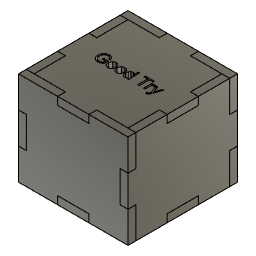
Box V2 v3 (Autodesk Fusion 360 design; units mm, degrees)
Autodesk Fusion 360 part; units mm, degrees
note: some values were not read from the file. Chosen so that the rebuilt part matches the saved one: which bodies a step acts on; the layout of a text.
sketch "Top-Bottom" plane through (0, 0, 0) normal (0, 0, 1) x (1, 0, 0)
  line L0 (0, 0) -> (30, 0)
  line L1 (30, 0) -> (30, 30)
  line L2 (30, 30) -> (0, 30)
  line L3 (0, 30) -> (0, 0)
  line L4 (-2.5, 20) -> (0, 20)
  line L5 (0, 20) -> (0, 10)
  line L6 (0, 10) -> (-2.5, 10)
  line L7 (-2.5, 10) -> (-2.5, 20)
  line L8 (15, 30) -> (15, 0) construction
  line L9 (0, 15) -> (30, 15) construction
  line L10 (10, 32.5) -> (20, 32.5)
  line L11 (20, 32.5) -> (20, 30)
  line L12 (20, 30) -> (10, 30)
  line L13 (10, 30) -> (10, 32.5)
  line L14 (20, 0) -> (10, 0)
  line L15 (10, 0) -> (10, -2.5)
  line L16 (20, -2.5) -> (20, 0)
  line L17 (10, -2.5) -> (20, -2.5)
  line L18 (30, 20) -> (30, 10)
  line L19 (30, 10) -> (32.5, 10)
  line L20 (32.5, 20) -> (30, 20)
  line L21 (32.5, 10) -> (32.5, 20)
  point P0 (15, 0)
  point P1 (30, 15)
  dimension "d4" = 30
  dimension "d5" = 30
  dimension "d9" = 2.5
  dimension "d10" = 10
  dimension "d11" = 10
  dimension "d12" = 2.5
  constraint horizontal L0
  constraint vertical L1
  constraint horizontal L2
  constraint vertical L3
  constraint coincident L0.start L3.end
  constraint horizontal L4
  constraint vertical L5
  constraint horizontal L6
  constraint vertical L7
  constraint midpoint L3 L5
  constraint midpoint L2 L8.start
  constraint midpoint L0 P0
  constraint midpoint L3 L9.start
  constraint midpoint L1 P1
  constraint horizontal L10
  constraint vertical L11
  constraint horizontal L12
  constraint vertical L13
  constraint midpoint L2 L12
  constraint symmetric L8.start L9 P0
  constraint symmetric L9 L10.start L15.end
  constraint symmetric L9 L10.end L16.start
  constraint symmetric L9 L11.end L14.start
  constraint symmetric L9 L12.end L14.end
  constraint symmetric L4.start L8 L20.start
  constraint symmetric L4.end L8 L18.start
  constraint symmetric L5.end L8 L18.end
  constraint symmetric L6.end L8 L19.end
  constraint symmetric L8 L9.start P1
  measures "d4" distance of L0.start L0.end
  measures "d5" distance of L0.start L2.end
  measures "d9" distance of L4.start L4.end
  measures "d10" distance of L4.start L6.end
  measures "d11" distance of L10.start L10.end
  measures "d12" distance of L10.start L12.end
extrude "Extrude1" add sketch "Top-Bottom" along normal blind 2.5 makes body 1
sketch "Front-Back" plane through (0, -2.5, 0) normal (0, -1, 0) x (1, 0, 0)
  line L0 (10, 0) -> (20, 0)
  line L1 (20, 0) -> (20, 2.5)
  line L2 (20, 2.5) -> (10, 2.5)
  line L3 (10, 2.5) -> (10, 0)
  line L4 (0, 0) -> (30, 0)
  line L5 (30, 0) -> (30, 30)
  line L6 (30, 30) -> (0, 30)
  line L7 (0, 30) -> (0, 0)
  line L8 (-2.5, 10) -> (0, 10)
  line L9 (0, 10) -> (0, 0)
  line L10 (0, 0) -> (-2.5, 0)
  line L11 (-2.5, 0) -> (-2.5, 10)
  line L12 (0, 20) -> (-2.5, 20)
  line L13 (-2.5, 30) -> (0, 30)
  line L14 (0, 30) -> (0, 20)
  line L15 (-2.5, 20) -> (-2.5, 30)
  line L16 (15, 30) -> (15, 0) construction
  line L17 (32.5, 30) -> (30, 30)
  line L18 (30, 20) -> (32.5, 20)
  line L19 (32.5, 20) -> (32.5, 30)
  line L20 (30, 30) -> (30, 20)
  line L21 (32.5, 0) -> (32.5, 10)
  line L22 (30, 0) -> (32.5, 0)
  line L23 (32.5, 10) -> (30, 10)
  line L24 (30, 10) -> (30, 0)
  point P0 (30, 30)
  point P1 (30, 0)
  point P2 (30, 0)
  dimension "d18" = 30
  dimension "d19" = 30
  dimension "d20" = 2.5
  dimension "d21" = 10
  dimension "d22" = 2.5
  dimension "d23" = 10
  constraint horizontal L4
  constraint vertical L5
  constraint horizontal L6
  constraint vertical L7
  constraint coincident L4.start L7.end
  constraint horizontal L8
  constraint vertical L9
  constraint horizontal L10
  constraint vertical L11
  constraint horizontal L13
  constraint vertical L14
  constraint horizontal L12
  constraint vertical L15
  constraint coincident L6.end L7.start
  constraint midpoint L6 L16.start
  constraint midpoint L4 L16.end
  constraint symmetric L4.start L16 P2
  constraint symmetric L6.end L16 P0
  constraint symmetric L8.start L16 L21.end
  constraint symmetric L8.end L16 L23.end
  constraint symmetric L10.end L16 L21.start
  constraint symmetric L13.start L16 L17.start
  constraint symmetric L12.start L16 L18.start
  constraint symmetric L12.end L16 L18.end
  measures "d18" distance of L4.start P2
  measures "d19" distance of L4.start L6.end
  measures "d20" distance of L8.start L8.end
  measures "d21" distance of L8.start L10.end
  measures "d22" distance of L13.start L6.end
  measures "d23" distance of L13.start L12.end
extrude "Extrude2" add sketch "Front-Back" against normal blind 2.5 separate body contours L1 L2 L3 L4 L5 L6 L7 L9 L14 L20 L24 | L7 L8 L9 L10 L11 | L5 L21 L22 L23 L24 | L7 L12 L13 L14 L15 | L5 L17 L18 L19 L20 makes body 2
ref_plane "WorkPlane1" through (15, 15, 15) normal (0, 0, -1) x (-1, 0, 0)
mirror "Mirror1" about plane through (15, 15, 15) normal (0, 0, -1) of bodies 1 makes body 3
ref_plane "WorkPlane2" through (15, 15, 15) normal (0, 1, 0) x (0, 0, 1)
mirror "Mirror2" about plane through (15, 15, 15) normal (0, 1, 0) of bodies 2 makes body 4
combine "Combine1" operation cut target body 2 tool bodies 3 keep tools
combine "Combine2" operation cut target body 4 tool bodies 3 keep tools
sketch "Left-Right" plane through (32.5, 0, 0) normal (1, 0, 0) x (0, 1, 0)
  line L0 (10, 0) -> (20, 0)
  line L1 (20, 0) -> (20, 2.5)
  line L2 (20, 2.5) -> (10, 2.5)
  line L3 (10, 2.5) -> (10, 0)
  line L4 (0, 0) -> (30, 0)
  line L5 (30, 0) -> (30, 30)
  line L6 (30, 30) -> (0, 30)
  line L7 (0, 30) -> (0, 0)
  line L8 (-2.5, 20) -> (0, 20)
  line L9 (0, 20) -> (0, 10)
  line L10 (0, 10) -> (-2.5, 10)
  line L11 (-2.5, 10) -> (-2.5, 20)
  line L12 (15, 30) -> (15, 0) construction
  line L13 (30, 10) -> (32.5, 10)
  line L14 (30, 20) -> (30, 10)
  line L15 (32.5, 10) -> (32.5, 20)
  line L16 (32.5, 20) -> (30, 20)
  dimension "d30" = 30
  dimension "d31" = 30
  dimension "d32" = 2.5
  dimension "d33" = 10
  constraint horizontal L4
  constraint vertical L5
  constraint horizontal L6
  constraint vertical L7
  constraint coincident L4.start L7.end
  constraint horizontal L8
  constraint vertical L9
  constraint horizontal L10
  constraint vertical L11
  constraint midpoint L7 L9
  constraint midpoint L6 L12.start
  constraint midpoint L4 L12.end
  constraint symmetric L8.start L12 L15.end
  constraint symmetric L8.end L12 L14.start
  constraint symmetric L9.end L12 L13.start
  constraint symmetric L10.end L12 L13.end
  measures "d30" distance of L4.start L4.end
  measures "d31" distance of L4.start L6.end
  measures "d32" distance of L8.start L8.end
  measures "d33" distance of L8.start L10.end
extrude "Extrude3" add sketch "Left-Right" against normal blind 2.5 separate body contours L1 L2 L3 L4 L5 L6 L7 L9 L14 | L7 L8 L9 L10 L11 | L5 L13 L14 L15 L16 makes body 5
combine "Combine3" operation cut target body 5 tool bodies 3 keep tools
ref_plane "WorkPlane3" through (15, 15, 15) normal (-1, 0, 0) x (0, 0, 1)
mirror "Mirror3" about plane through (15, 15, 15) normal (-1, 0, 0) of bodies 5 makes body 6
sketch "Text-Top" plane through (0, 0, 30) normal (0, 0, 1) x (-1, 0, 0)
  line L0 (0, -10) -> (0, 0)
  line L1 (0, 0) -> (-10, 0)
  line L2 (-10, 0) -> (-10, 2.5)
  line L3 (-10, 2.5) -> (-20, 2.5)
  line L4 (-20, 2.5) -> (-20, 0)
  line L5 (-20, 0) -> (-30, 0)
  line L6 (-30, 0) -> (-30, -10)
  line L7 (-30, -10) -> (-32.5, -10)
  line L8 (-32.5, -10) -> (-32.5, -20)
  line L9 (-32.5, -20) -> (-30, -20)
  line L10 (-30, -20) -> (-30, -30)
  line L11 (-30, -30) -> (-20, -30)
  line L12 (-20, -30) -> (-20, -32.5)
  line L13 (-20, -32.5) -> (-10, -32.5)
  line L14 (-10, -32.5) -> (-10, -30)
  line L15 (-10, -30) -> (0, -30)
  line L16 (0, -30) -> (0, -20)
  line L17 (0, -20) -> (2.5, -20)
  line L18 (2.5, -20) -> (2.5, -10)
  line L19 (2.5, -10) -> (0, -10)
  line L20 (-5, -12.5) -> (-25, -12.5) construction
  line L21 (-25, -12.5) -> (-25, -17.5) construction
  line L22 (-25, -17.5) -> (-5, -17.5) construction
  line L23 (-5, -17.5) -> (-5, -12.5) construction
  line L24 (2.5, -15) -> (-5, -15) construction
  line L25 (-25, -15) -> (-32.5, -15) construction
  dimension "d39" = 5
  dimension "d42" = 7.5
  dimension "d43" = 7.5
  text T0 "Good Try" font "Arial" height 5 align ink ink in box 0 x 0 at (-5.01, -12.52) x (-1, 0) y (0, -1) spacing 1 kerned height is em
  constraint perpendicular L20 L21
  constraint parallel L20 L22
  constraint parallel L21 L23
  constraint midpoint L18 L24.start
  constraint perpendicular L18 L24
  constraint midpoint L23 L24.end
  constraint midpoint L21 L25.start
  constraint midpoint L8 L25.end
  constraint perpendicular L8 L25
  measures "d39" distance of L20.end L21.end
  measures "d42" distance of L24.start L24.end
  measures "d43" distance of L25.start L25.end
extrude "Extrude4" cut sketch "Text-Top" against normal blind 2.5 text T0 bodies 3 makes body 7 at (12.6268, 15.5251, 30) makes body 8 at (15.3464, 15.5191, 30) makes body 9 at (15.1604, 4.5046, 30)
delete_body "RemoveBody1" bodies 3
delete_body "RemoveBody2" bodies 7
delete_body "RemoveBody3" bodies 8
sketch "Final-Top" plane through (0, 0, 30) normal (0, 0, 1) x (-1, 0, 0)
  line L0 (0, -10) -> (0, 0)
  line L1 (0, 0) -> (-10, 0)
  line L2 (-10, 0) -> (-10, 2.5)
  line L3 (-10, 2.5) -> (-20, 2.5)
  line L4 (-20, 2.5) -> (-20, 0)
  line L5 (-20, 0) -> (-30, 0)
  line L6 (-30, 0) -> (-30, -10)
  line L7 (-30, -10) -> (-32.5, -10)
  line L8 (-32.5, -10) -> (-32.5, -20)
  line L9 (-32.5, -20) -> (-30, -20)
  line L10 (-30, -20) -> (-30, -30)
  line L11 (-30, -30) -> (-20, -30)
  line L12 (-20, -30) -> (-20, -32.5)
  line L13 (-20, -32.5) -> (-10, -32.5)
  line L14 (-10, -32.5) -> (-10, -30)
  line L15 (-10, -30) -> (0, -30)
  line L16 (0, -30) -> (0, -20)
  line L17 (0, -20) -> (2.5, -20)
  line L18 (2.5, -20) -> (2.5, -10)
  line L19 (2.5, -10) -> (0, -10)
  line L20 (-7.8567, -14.3096) -> (-7.8567, -14.9761)
  line L21 (-7.8567, -14.9761) -> (-6.8044, -14.9761)
  line L22 (-6.8044, -14.9761) -> (-6.8044, -15.396)
  line L23 (-6.8044, -15.396) -> (-8.3205, -15.3984)
  line L24 (-8.3205, -15.3984) -> (-8.3205, -14.0703)
  spline S0 degree 3 poles (-8.3205, -14.0703) (-8.2052, -13.984) (-7.9813, -13.8165) (-7.7248, -13.7055) (-7.6003, -13.6516) knots 0 0 0 0 0.043036 0.083562 0.083562 0.083562 0.083562
  spline S1 degree 3 poles (-7.6003, -13.6516) (-7.4761, -13.6106) (-7.2286, -13.5291) (-6.9683, -13.5172) (-6.8386, -13.5112) knots 0 0 0 0 0.039044 0.077778 0.077778 0.077778 0.077778
  spline S2 degree 3 poles (-6.8386, -13.5112) (-6.6684, -13.5198) (-6.3351, -13.5366) (-6.0298, -13.6712) (-5.8804, -13.737) knots 0 0 0 0 0.050639 0.099191 0.099191 0.099191 0.099191
  spline S3 degree 3 poles (-5.8804, -13.737) (-5.7456, -13.8205) (-5.4771, -13.9868) (-5.312, -14.256) (-5.2297, -14.3901) knots 0 0 0 0 0.046824 0.093334 0.093334 0.093334 0.093334
  spline S4 degree 3 poles (-5.2297, -14.3901) (-5.1657, -14.5387) (-5.0343, -14.8434) (-5.0182, -15.1749) (-5.01, -15.3447) knots 0 0 0 0 0.048136 0.098667 0.098667 0.098667 0.098667
  spline S5 degree 3 poles (-5.01, -15.3447) (-5.0187, -15.5152) (-5.036, -15.8528) (-5.1648, -16.1653) (-5.2285, -16.32) knots 0 0 0 0 0.050801 0.100602 0.100602 0.100602 0.100602
  spline S6 degree 3 poles (-5.2285, -16.32) (-5.3078, -16.4605) (-5.4633, -16.7356) (-5.7277, -16.9082) (-5.8572, -16.9927) knots 0 0 0 0 0.047611 0.093274 0.093274 0.093274 0.093274
  spline S7 degree 3 poles (-5.8572, -16.9927) (-6.0021, -17.0567) (-6.3029, -17.1897) (-6.6316, -17.2046) (-6.802, -17.2124) knots 0 0 0 0 0.047105 0.097758 0.097758 0.097758 0.097758
  spline S8 degree 3 poles (-6.802, -17.2124) (-6.9263, -17.2079) (-7.1663, -17.1993) (-7.3941, -17.1233) (-7.5039, -17.0867) knots 0 0 0 0 0.03709 0.071636 0.071636 0.071636 0.071636
  spline S9 degree 3 poles (-7.5039, -17.0867) (-7.6014, -17.0424) (-7.7884, -16.9575) (-7.9287, -16.8079) (-7.9958, -16.7363) knots 0 0 0 0 0.031773 0.060917 0.060917 0.060917 0.060917
  spline S10 degree 3 poles (-7.9958, -16.7363) (-8.0526, -16.6521) (-8.1743, -16.4716) (-8.2346, -16.2622) (-8.2668, -16.1504) knots 0 0 0 0 0.030262 0.06491 0.06491 0.06491 0.06491
  line L25 (-8.2668, -16.1504) -> (-7.8396, -16.0332)
  spline S11 degree 3 poles (-7.8396, -16.0332) (-7.8133, -16.1164) (-7.7653, -16.2685) (-7.6787, -16.4023) (-7.6394, -16.4629) knots 0 0 0 0 0.026032 0.047595 0.047595 0.047595 0.047595
  spline S12 degree 3 poles (-7.6394, -16.4629) (-7.5934, -16.5131) (-7.4964, -16.6192) (-7.3662, -16.6807) (-7.2976, -16.7131) knots 0 0 0 0 0.020222 0.042723 0.042723 0.042723 0.042723
  spline S13 degree 3 poles (-7.2976, -16.7131) (-7.2202, -16.7405) (-7.0607, -16.797) (-6.8916, -16.8037) (-6.8044, -16.8071) knots 0 0 0 0 0.024475 0.05046 0.05046 0.05046 0.05046
  spline S14 degree 3 poles (-6.8044, -16.8071) (-6.7026, -16.8041) (-6.5104, -16.7984) (-6.3284, -16.737) (-6.2429, -16.7082) knots 0 0 0 0 0.030374 0.057295 0.057295 0.057295 0.057295
  spline S15 degree 3 poles (-6.2429, -16.7082) (-6.1689, -16.6739) (-6.0272, -16.6082) (-5.9147, -16.5) (-5.8608, -16.4482) knots 0 0 0 0 0.024261 0.046502 0.046502 0.046502 0.046502
  spline S16 degree 3 poles (-5.8608, -16.4482) (-5.8152, -16.3935) (-5.7249, -16.2851) (-5.6648, -16.1574) (-5.635, -16.0942) knots 0 0 0 0 0.021272 0.042143 0.042143 0.042143 0.042143
  spline S17 degree 3 poles (-5.635, -16.0942) (-5.5951, -15.98) (-5.5138, -15.7468) (-5.5035, -15.4999) (-5.4983, -15.374) knots 0 0 0 0 0.036094 0.073664 0.073664 0.073664 0.073664
  spline S18 degree 3 poles (-5.4983, -15.374) (-5.5029, -15.2256) (-5.5116, -14.9487) (-5.6151, -14.6922) (-5.6631, -14.5732) knots 0 0 0 0 0.044138 0.082326 0.082326 0.082326 0.082326
  spline S19 degree 3 poles (-5.6631, -14.5732) (-5.7238, -14.4729) (-5.8444, -14.2739) (-6.0439, -14.1541) (-6.1428, -14.0947) knots 0 0 0 0 0.034607 0.068675 0.068675 0.068675 0.068675
  spline S20 degree 3 poles (-6.1428, -14.0947) (-6.2495, -14.0491) (-6.4633, -13.9578) (-6.6955, -13.9449) (-6.8118, -13.9385) knots 0 0 0 0 0.034521 0.069165 0.069165 0.069165 0.069165
  spline S21 degree 3 poles (-6.8118, -13.9385) (-6.914, -13.9435) (-7.12, -13.9537) (-7.3144, -14.0223) (-7.4123, -14.0569) knots 0 0 0 0 0.030539 0.061503 0.061503 0.061503 0.061503
  spline S22 degree 3 poles (-7.4123, -14.0569) (-7.5004, -14.0939) (-7.6588, -14.1604) (-7.7958, -14.2637) (-7.8567, -14.3096) knots 0 0 0 0 0.028516 0.05129 0.05129 0.05129 0.05129
  spline S23 degree 3 poles (-12.7956, -13.5137) (-12.6249, -13.5262) (-12.2942, -13.5504) (-12.0389, -13.761) (-11.9155, -13.8628) knots 0 0 0 0 0.049993 0.096791 0.096791 0.096791 0.096791
  spline S24 degree 3 poles (-11.9155, -13.8628) (-11.8178, -13.9999) (-11.6044, -14.2994) (-11.5884, -14.6685) (-11.5798, -14.8686) knots 0 0 0 0 0.049486 0.108074 0.108074 0.108074 0.108074
  spline S25 degree 3 poles (-11.5798, -14.8686) (-11.5898, -15.0869) (-11.6083, -15.4883) (-11.8637, -15.7954) (-11.9802, -15.9355) knots 0 0 0 0 0.063477 0.116753 0.116753 0.116753 0.116753
  spline S26 degree 3 poles (-11.9802, -15.9355) (-12.0996, -16.0195) (-12.3442, -16.1916) (-12.6428, -16.2128) (-12.7956, -16.2236) knots 0 0 0 0 0.042941 0.087955 0.087955 0.087955 0.087955
  spline S27 degree 3 poles (-12.7956, -16.2236) (-12.9642, -16.2106) (-13.2927, -16.1852) (-13.5462, -15.9754) (-13.6697, -15.8733) knots 0 0 0 0 0.049367 0.096242 0.096242 0.096242 0.096242
  spline S28 degree 3 poles (-13.6697, -15.8733) (-13.7685, -15.7393) (-13.9801, -15.4527) (-13.999, -15.0955) (-14.009, -14.9053) knots 0 0 0 0 0.048869 0.104602 0.104602 0.104602 0.104602
  spline S29 degree 3 poles (-14.009, -14.9053) (-14.0061, -14.7543) (-14.0008, -14.4827) (-13.9025, -14.2301) (-13.8589, -14.1179) knots 0 0 0 0 0.044866 0.080708 0.080708 0.080708 0.080708
  spline S30 degree 3 poles (-13.8589, -14.1179) (-13.803, -14.0275) (-13.6908, -13.8462) (-13.5117, -13.7304) (-13.4219, -13.6723) knots 0 0 0 0 0.03145 0.063109 0.063109 0.063109 0.063109
  spline S31 degree 3 poles (-13.4219, -13.6723) (-13.3236, -13.6261) (-13.1251, -13.5326) (-12.9061, -13.52) (-12.7956, -13.5137) knots 0 0 0 0 0.032274 0.065137 0.065137 0.065137 0.065137
  line L26 (-16.614, -17.1513) -> (-16.614, -13.5722)
  line L27 (-16.614, -13.5722) -> (-16.2063, -13.5722)
  line L28 (-16.2063, -13.5722) -> (-16.2063, -13.8994)
  spline S32 degree 3 poles (-16.2063, -13.8994) (-16.1134, -13.7869) (-15.9251, -13.5588) (-15.6305, -13.5288) (-15.4812, -13.5137) knots 0 0 0 0 0.042007 0.085152 0.085152 0.085152 0.085152
  spline S33 degree 3 poles (-15.4812, -13.5137) (-15.3799, -13.5208) (-15.1771, -13.5351) (-14.9998, -13.6347) (-14.9111, -13.6846) knots 0 0 0 0 0.03006 0.060176 0.060176 0.060176 0.060176
  spline S34 degree 3 poles (-14.9111, -13.6846) (-14.8288, -13.7482) (-14.6606, -13.8785) (-14.5598, -14.066) (-14.5083, -14.1618) knots 0 0 0 0 0.030848 0.063081 0.063081 0.063081 0.063081
  spline S35 degree 3 poles (-14.5083, -14.1618) (-14.4667, -14.2704) (-14.3797, -14.497) (-14.3703, -14.7397) (-14.3655, -14.8662) knots 0 0 0 0 0.034627 0.072303 0.072303 0.072303 0.072303
  spline S36 degree 3 poles (-14.3655, -14.8662) (-14.3701, -14.9907) (-14.3791, -15.2319) (-14.4571, -15.4602) (-14.4949, -15.5705) knots 0 0 0 0 0.037159 0.071956 0.071956 0.071956 0.071956
  spline S37 degree 3 poles (-14.4949, -15.5705) (-14.5422, -15.669) (-14.6343, -15.8606) (-14.8016, -15.9915) (-14.883, -16.0552) knots 0 0 0 0 0.03227 0.062841 0.062841 0.062841 0.062841
  spline S38 degree 3 poles (-14.883, -16.0552) (-14.9723, -16.1043) (-15.1526, -16.2035) (-15.358, -16.2169) (-15.4617, -16.2236) knots 0 0 0 0 0.030177 0.060923 0.060923 0.060923 0.060923
  spline S39 degree 3 poles (-15.4617, -16.2236) (-15.5366, -16.22) (-15.6821, -16.2131) (-15.8148, -16.1536) (-15.8791, -16.1247) knots 0 0 0 0 0.022293 0.043242 0.043242 0.043242 0.043242
  spline S40 degree 3 poles (-15.8791, -16.1247) (-15.937, -16.0897) (-16.051, -16.0208) (-16.1354, -15.9178) (-16.177, -15.8672) knots 0 0 0 0 0.020129 0.039633 0.039633 0.039633 0.039633
  line L29 (-16.177, -15.8672) -> (-16.177, -17.1513)
  line L30 (-16.177, -17.1513) -> (-16.614, -17.1513)
  line L31 (-21.907, -14.9297) -> (-21.907, -13.5722)
  line L32 (-21.907, -13.5722) -> (-21.4675, -13.5722)
  line L33 (-21.4675, -13.5722) -> (-21.4675, -16.165)
  line L34 (-21.4675, -16.165) -> (-21.863, -16.165)
  line L35 (-21.863, -16.165) -> (-21.863, -15.772)
  spline S41 degree 3 poles (-21.863, -15.772) (-21.9071, -15.8518) (-21.982, -15.9877) (-22.0957, -16.0925) (-22.1426, -16.1357) knots 0 0 0 0 0.027125 0.046136 0.046136 0.046136 0.046136
  spline S42 degree 3 poles (-22.1426, -16.1357) (-22.1863, -16.1614) (-22.2735, -16.2125) (-22.3743, -16.2199) (-22.4246, -16.2236) knots 0 0 0 0 0.014986 0.029889 0.029889 0.029889 0.029889
  spline S43 degree 3 poles (-22.4246, -16.2236) (-22.5007, -16.2166) (-22.6611, -16.2018) (-22.8021, -16.1233) (-22.8762, -16.082) knots 0 0 0 0 0.022678 0.047799 0.047799 0.047799 0.047799
  line L36 (-22.8762, -16.082) -> (-22.7248, -15.6743)
  spline S44 degree 3 poles (-22.7248, -15.6743) (-22.6723, -15.7021) (-22.5711, -15.7555) (-22.4573, -15.765) (-22.4026, -15.7695) knots 0 0 0 0 0.017625 0.033913 0.033913 0.033913 0.033913
  spline S45 degree 3 poles (-22.4026, -15.7695) (-22.3558, -15.7659) (-22.2623, -15.7587) (-22.1833, -15.7081) (-22.1438, -15.6828) knots 0 0 0 0 0.013843 0.027672 0.027672 0.027672 0.027672
  spline S46 degree 3 poles (-22.1438, -15.6828) (-22.1081, -15.6504) (-22.0343, -15.5835) (-21.9986, -15.4904) (-21.9802, -15.4424) knots 0 0 0 0 0.014269 0.029448 0.029448 0.029448 0.029448
  spline S47 degree 3 poles (-21.9802, -15.4424) (-21.9589, -15.361) (-21.9147, -15.193) (-21.9096, -15.0193) (-21.907, -14.9297) knots 0 0 0 0 0.025144 0.05194 0.05194 0.05194 0.05194
  line L37 (-20.0442, -16.729) -> (-20.0442, -13.5722)
  line L38 (-20.0442, -13.5722) -> (-19.5705, -13.5722)
  line L39 (-19.5705, -13.5722) -> (-19.5705, -16.729)
  line L40 (-19.5705, -16.729) -> (-18.3913, -16.729)
  line L41 (-18.3913, -16.729) -> (-18.3913, -17.1513)
  line L42 (-18.3913, -17.1513) -> (-21.2283, -17.1513)
  line L43 (-21.2283, -17.1513) -> (-21.2283, -16.729)
  line L44 (-21.2283, -16.729) -> (-20.0442, -16.729)
  spline S48 degree 3 poles (-23.7624, -12.6213) (-23.7083, -12.5918) (-23.5958, -12.5304) (-23.4676, -12.5235) (-23.4011, -12.52) knots 0 0 0 0 0.018258 0.037953 0.037953 0.037953 0.037953
  spline S49 degree 3 poles (-23.4011, -12.52) (-23.356, -12.5228) (-23.2594, -12.5287) (-23.1671, -12.5581) (-23.1179, -12.5737) knots 0 0 0 0 0.013495 0.028922 0.028922 0.028922 0.028922
  line L45 (-23.1179, -12.5737) -> (-23.0691, -12.9863)
  spline S50 degree 3 poles (-23.0691, -12.9863) (-23.1138, -12.9749) (-23.1964, -12.9539) (-23.2815, -12.9493) (-23.3205, -12.9472) knots 0 0 0 0 0.013803 0.025502 0.025502 0.025502 0.025502
  spline S51 degree 3 poles (-23.3205, -12.9472) (-23.3651, -12.9484) (-23.4464, -12.9504) (-23.5212, -12.9819) (-23.5549, -12.9961) knots 0 0 0 0 0.01324 0.024128 0.024128 0.024128 0.024128
  spline S52 degree 3 poles (-23.5549, -12.9961) (-23.583, -13.0141) (-23.6397, -13.0505) (-23.6791, -13.1052) (-23.699, -13.1328) knots 0 0 0 0 0.009913 0.020017 0.020017 0.020017 0.020017
  spline S53 degree 3 poles (-23.699, -13.1328) (-23.7176, -13.1708) (-23.7697, -13.2767) (-23.8084, -13.3884) (-23.8332, -13.4599) knots 0 0 0 0 0.012695 0.035391 0.035391 0.035391 0.035391
  spline S54 degree 3 poles (-23.8332, -13.4599) (-23.8385, -13.475) (-23.851, -13.511) (-23.8645, -13.5467) (-23.8723, -13.5674) knots 0 0 0 0 0.004787 0.011431 0.011431 0.011431 0.011431
  line L46 (-23.8723, -13.5674) -> (-22.8884, -16.165)
  line L47 (-22.8884, -16.165) -> (-23.3621, -16.165)
  line L48 (-23.3621, -16.165) -> (-23.9016, -14.6636)
  spline S55 degree 3 poles (-23.9016, -14.6636) (-23.9359, -14.5663) (-24.0057, -14.3683) (-24.0613, -14.1659) (-24.0896, -14.063) knots 0 0 0 0 0.03094 0.06295 0.06295 0.06295 0.06295
  spline S56 degree 3 poles (-24.0896, -14.063) (-24.116, -14.1631) (-24.1685, -14.3624) (-24.2364, -14.5569) (-24.2703, -14.6538) knots 0 0 0 0 0.031038 0.061804 0.061804 0.061804 0.061804
  line L49 (-24.2703, -14.6538) -> (-24.8245, -16.165)
  line L50 (-24.8245, -16.165) -> (-25.2639, -16.165)
  line L51 (-25.2639, -16.165) -> (-24.2776, -13.5283)
  spline S57 degree 3 poles (-24.2776, -13.5283) (-24.2328, -13.4071) (-24.159, -13.2074) (-24.0671, -13.0154) (-24.031, -12.9399) knots 0 0 0 0 0.038729 0.063825 0.063825 0.063825 0.063825
  spline S58 degree 3 poles (-24.031, -12.9399) (-23.9928, -12.8739) (-23.922, -12.7516) (-23.8128, -12.6624) (-23.7624, -12.6213) knots 0 0 0 0 0.022641 0.041975 0.041975 0.041975 0.041975
  spline S59 degree 3 poles (-10.0149, -13.5137) (-9.8441, -13.5262) (-9.5134, -13.5504) (-9.2582, -13.761) (-9.1348, -13.8628) knots 0 0 0 0 0.049993 0.096791 0.096791 0.096791 0.096791
  spline S60 degree 3 poles (-9.1348, -13.8628) (-9.037, -13.9999) (-8.8236, -14.2994) (-8.8077, -14.6685) (-8.7991, -14.8686) knots 0 0 0 0 0.049486 0.108074 0.108074 0.108074 0.108074
  spline S61 degree 3 poles (-8.7991, -14.8686) (-8.8091, -15.0869) (-8.8275, -15.4883) (-9.0829, -15.7954) (-9.1995, -15.9355) knots 0 0 0 0 0.063477 0.116753 0.116753 0.116753 0.116753
  spline S62 degree 3 poles (-9.1995, -15.9355) (-9.3189, -16.0195) (-9.5634, -16.1916) (-9.8621, -16.2128) (-10.0149, -16.2236) knots 0 0 0 0 0.042941 0.087955 0.087955 0.087955 0.087955
  spline S63 degree 3 poles (-10.0149, -16.2236) (-10.1834, -16.2106) (-10.512, -16.1852) (-10.7654, -15.9754) (-10.8889, -15.8733) knots 0 0 0 0 0.049367 0.096242 0.096242 0.096242 0.096242
  spline S64 degree 3 poles (-10.8889, -15.8733) (-10.9878, -15.7393) (-11.1994, -15.4527) (-11.2182, -15.0955) (-11.2283, -14.9053) knots 0 0 0 0 0.048869 0.104602 0.104602 0.104602 0.104602
  spline S65 degree 3 poles (-11.2283, -14.9053) (-11.2253, -14.7543) (-11.2201, -14.4827) (-11.1218, -14.2301) (-11.0781, -14.1179) knots 0 0 0 0 0.044866 0.080708 0.080708 0.080708 0.080708
  spline S66 degree 3 poles (-11.0781, -14.1179) (-11.0222, -14.0275) (-10.91, -13.8462) (-10.7309, -13.7304) (-10.6411, -13.6723) knots 0 0 0 0 0.03145 0.063109 0.063109 0.063109 0.063109
  spline S67 degree 3 poles (-10.6411, -13.6723) (-10.5428, -13.6261) (-10.3444, -13.5326) (-10.1254, -13.52) (-10.0149, -13.5137) knots 0 0 0 0 0.032274 0.065137 0.065137 0.065137 0.065137
sketch "Final-Bottom" plane through (0, 0, 2.5) normal (0, 0, 1) x (-1, 0, 0)
  line L0 (0, -10) -> (0, 0)
  line L1 (0, 0) -> (-10, 0)
  line L2 (-10, 0) -> (-10, 2.5)
  line L3 (-10, 2.5) -> (-20, 2.5)
  line L4 (-20, 2.5) -> (-20, 0)
  line L5 (-20, 0) -> (-30, 0)
  line L6 (-30, 0) -> (-30, -10)
  line L7 (-30, -10) -> (-32.5, -10)
  line L8 (-32.5, -10) -> (-32.5, -20)
  line L9 (-32.5, -20) -> (-30, -20)
  line L10 (-30, -20) -> (-30, -30)
  line L11 (-30, -30) -> (-20, -30)
  line L12 (-20, -30) -> (-20, -32.5)
  line L13 (-20, -32.5) -> (-10, -32.5)
  line L14 (-10, -32.5) -> (-10, -30)
  line L15 (-10, -30) -> (0, -30)
  line L16 (0, -30) -> (0, -20)
  line L17 (0, -20) -> (2.5, -20)
  line L18 (2.5, -20) -> (2.5, -10)
  line L19 (2.5, -10) -> (0, -10)
sketch "Final-Front-Back" plane through (0, -2.5, 0) normal (0, -1, 0) x (1, 0, 0)
  line L0 (10, 27.5) -> (10, 30)
  line L1 (10, 30) -> (-2.5, 30)
  line L2 (-2.5, 30) -> (-2.5, 20)
  line L3 (-2.5, 20) -> (0, 20)
  line L4 (0, 20) -> (0, 10)
  line L5 (0, 10) -> (-2.5, 10)
  line L6 (-2.5, 10) -> (-2.5, 0)
  line L7 (-2.5, 0) -> (10, 0)
  line L8 (10, 0) -> (10, 2.5)
  line L9 (10, 2.5) -> (20, 2.5)
  line L10 (20, 2.5) -> (20, 0)
  line L11 (20, 0) -> (32.5, 0)
  line L12 (32.5, 0) -> (32.5, 10)
  line L13 (32.5, 10) -> (30, 10)
  line L14 (30, 10) -> (30, 20)
  line L15 (30, 20) -> (32.5, 20)
  line L16 (32.5, 20) -> (32.5, 30)
  line L17 (32.5, 30) -> (20, 30)
  line L18 (20, 30) -> (20, 27.5)
  line L19 (20, 27.5) -> (10, 27.5)
sketch "Final-Left-Right" plane through (32.5, 0, 0) normal (1, 0, 0) x (0, 1, 0)
  line L0 (10, 27.5) -> (10, 30)
  line L1 (10, 30) -> (0, 30)
  line L2 (0, 30) -> (0, 20)
  line L3 (0, 20) -> (-2.5, 20)
  line L4 (-2.5, 20) -> (-2.5, 10)
  line L5 (-2.5, 10) -> (0, 10)
  line L6 (0, 10) -> (0, 0)
  line L7 (0, 0) -> (10, 0)
  line L8 (10, 0) -> (10, 2.5)
  line L9 (10, 2.5) -> (20, 2.5)
  line L10 (20, 2.5) -> (20, 0)
  line L11 (20, 0) -> (30, 0)
  line L12 (30, 0) -> (30, 10)
  line L13 (30, 10) -> (32.5, 10)
  line L14 (32.5, 10) -> (32.5, 20)
  line L15 (32.5, 20) -> (30, 20)
  line L16 (30, 20) -> (30, 30)
  line L17 (30, 30) -> (20, 30)
  line L18 (20, 30) -> (20, 27.5)
  line L19 (20, 27.5) -> (10, 27.5)
equation "len = 30 mm"
equation "wid = 2.5 mm"
equation "hei = 30 mm"
equation "d4 = hei"
equation "d5 = len"
equation "slot = 10 mm"
equation "nslot = len / slot"
equation "d9 = wid"
equation "d10 = slot"
equation "d11 = slot"
equation "d12 = wid"
equation "thick = wid"
equation "d14 = thick"
equation "d18 = len"
equation "d19 = hei"
equation "d20 = wid"
equation "d21 = slot"
equation "d22 = wid"
equation "d23 = slot"
equation "d24 = -wid"
equation "d26 = -len / 2"
equation "d28 = len / 2"
equation "d30 = hei"
equation "d31 = len"
equation "d32 = wid"
equation "d33 = slot"
equation "d34 = -wid"
equation "d36 = len / 2"
equation "texth = 5 mm"
equation "d39 = texth"
equation "textl = len - textc"
equation "textc = wid + 5 mm"
equation "d42 = textc"
equation "d43 = textc"
equation "d44 = -wid"
named bodies: "Bottom", "Front", "Back", "Left", "Right", "Top"
